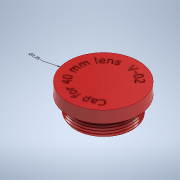
# Autodesk Inventor part: CapForSvBonyPlosse-40mm-V02
Saved by Autodesk Inventor 2021.1 (Build 251245010, 245A)
## iProperties
Created: 2020-10-08
Part Number: CapForSvBonyPlosse-40mm-V02
Material: PC/ABS Plastic
Document SubType Name: Modeling
Designer: robst
Density: 0.357273 g/cm^3
Appearance: Red
Author: robst
Autodesk Inventor part; units mm, degrees
ref_plane "YZ Plane" through (0, 0, 0) normal (1, 0, 0) x (0, 1, 0)
ref_plane "XZ Plane" through (0, 0, 0) normal (0, 1, 0) x (-1, 0, 0)
ref_plane "XY Plane" through (0, 0, 0) normal (0, 0, 1) x (1, 0, 0)
sketch "Sketch7" plane through (0, 0, 0) normal (0, 0, 1) x (1, 0, 0)
  line L0 (0, 0) -> (23.5712, 0)
  line L1 (23.5712, 0) -> (23.5712, 12.7)
  line L2 (23.5712, 12.7) -> (28.575, 12.7)
  line L3 (28.575, 12.7) -> (28.575, 22.225)
  line L4 (28.575, 22.225) -> (0, 22.225)
  line L5 (23.5712, 0) -> (20.3962, 0)
  line L6 (20.3962, 0) -> (20.3962, 19.05)
  line L7 (20.3962, 19.05) -> (0, 19.05)
  line L8 (0, 22.225) -> (0, 19.05)
  line L9 (0, -4.445) -> (0, 26.67) projected
  dimension "d71" = 9.525
  dimension "d72" = 12.7
  dimension "d73" = 23.5712
  dimension "d78" = 3.175
  dimension "d117" = 20.3962
  dimension "d118" = 28.575
  constraints: 18 end point, 5 perpendicular, 2 vertical, 1 horizontal, 1 point on line
  measures "d71" distance between parallel lines of L4 L2
  measures "d72" distance from line of L2 L0.start
  measures "d73" distance of L0.start L0.end
  measures "d78" distance between parallel lines of L1 L6
  measures "d117" distance between parallel lines of L6 L9
  measures "d118" distance from line of L3 L0.start
revolve "Revolution3" add sketch "Sketch7" angle 360 about axis through (0, -10, 0) along (0, 1, 0) contours L6 L7 L8 L4 L3 L2 L1 L0
sketch "Sketch10" plane through (0, 0, 0) normal (0, 0, 1) x (1, 0, 0)
  line L0 (23.5712, 12.7) -> (23.5712, 0) projected
  line L1 (23.5712, -2.1167) -> (23.5712, -4.0025)
  line L2 (23.5712, -4.0025) -> (22.3266, -3.284)
  line L3 (22.3266, -2.8352) -> (23.5712, -2.1167)
  line L4 (-23.5712, 0) -> (23.5712, 0) projected
  arc A0 (22.3266, -2.8352) -> (22.3266, -3.284) centre (22.4561, -3.0596) ccw
  line L5 (0, -7.3431) -> (0, 16.0405) projected
  point P0 (0, 0)
  dimension "d100" = 60
  dimension "d101" = 2.1167
  dimension "d102" = 0.2591
  dimension "d103" = 22.1971
  constraints: 6 end point, 2 point on circle, 2 tangent, 1 centre point, 1 collinear, 1 equal length, 1 vertical
  measures "d100" angle of L3 L2
  measures "d101" distance from line of L1.start L4
  measures "d102" radius of A0
  measures "d103" distance edge to line of A0 L5
coil "Coil6" sketch "Sketch10" operation cut axis through (0, -10, 0) along (0, 1, 0) pitch 2.1167 turns 8 hand right
sketch "Sketch11" plane through (0, 22.225, 0) normal (0, 1, 0) x (1, 0, 0)
  circle A0 centre (0, 0) radius 20.955 construction
  circle A1 centre (0, 0) radius 28.575 projected
  spline S0 degree 2 poles (12.0651, -13.3596) (12.4681, -12.9769) (13.4081, -12.6015) (13.915, -12.6375) knots 0 0 0 1 2 2 2
  spline S1 degree 2 poles (13.915, -12.6375) (14.4186, -12.6701) (15.4561, -13.2177) (15.9536, -13.7416) knots 0 0 0 1 2 2 2
  spline S2 degree 2 poles (15.9536, -13.7416) (16.4479, -14.2621) (16.9162, -15.2864) (16.9354, -15.8111) knots 0 0 0 1 2 2 2
  spline S3 degree 2 poles (16.9354, -15.8111) (16.9516, -16.3258) (16.5507, -17.2622) (16.131, -17.6609) knots 0 0 0 1 2 2 2
  spline S4 degree 2 poles (16.131, -17.6609) (15.9228, -17.8586) (15.4993, -18.1458) (15.3002, -18.2455) knots 0 0 0 1 2 2 2
  spline S5 degree 2 poles (15.3002, -18.2455) (15.1244, -18.3294) (14.7277, -18.4699) (14.5198, -18.5268) knots 0 0 0 1 2 2 2
  line L0 (14.5198, -18.5268) -> (13.8883, -17.8618)
  line L1 (13.8883, -17.8618) -> (13.932, -17.8204)
  spline S6 degree 2 poles (13.932, -17.8204) (14.0697, -17.8174) (14.4766, -17.7886) (14.7273, -17.723) knots 0 0 0 1 2 2 2
  spline S7 degree 2 poles (14.7273, -17.723) (14.968, -17.6604) (15.446, -17.4172) (15.6878, -17.1875) knots 0 0 0 1 2 2 2
  spline S8 degree 2 poles (15.6878, -17.1875) (15.9531, -16.9356) (16.2193, -16.2676) (16.1996, -15.8904) knots 0 0 0 1 2 2 2
  spline S9 degree 2 poles (16.1996, -15.8904) (16.1733, -15.513) (15.7589, -14.6866) (15.3793, -14.287) knots 0 0 0 1 2 2 2
  spline S10 degree 2 poles (15.3793, -14.287) (14.9743, -13.8605) (14.1858, -13.4405) (13.8069, -13.398) knots 0 0 0 1 2 2 2
  spline S11 degree 2 poles (13.8069, -13.398) (13.4377, -13.359) (12.7732, -13.5941) (12.5113, -13.8428) knots 0 0 0 1 2 2 2
  spline S12 degree 2 poles (12.5113, -13.8428) (12.2729, -14.0693) (11.9781, -14.5727) (11.9032, -14.8099) knots 0 0 0 1 2 2 2
  spline S13 degree 2 poles (11.9032, -14.8099) (11.835, -15.0408) (11.7823, -15.4358) (11.7791, -15.5602) knots 0 0 0 1 2 2 2
  line L2 (11.7791, -15.5602) -> (11.7388, -15.5984)
  line L3 (11.7388, -15.5984) -> (11.1137, -14.9402)
  spline S14 degree 2 poles (11.1137, -14.9402) (11.1907, -14.7457) (11.3209, -14.3985) (11.4411, -14.1821) knots 0 0 0 1 2 2 2
  spline S15 degree 2 poles (11.4411, -14.1821) (11.5651, -13.9495) (11.8166, -13.5956) (12.0651, -13.3596) knots 0 0 0 1 2 2 2
  spline S16 degree 2 poles (8.4215, -16.5515) (8.466, -16.4517) (8.6094, -16.104) (8.6959, -15.975) knots 0 0 0 1 2 2 2
  spline S17 degree 2 poles (8.6959, -15.975) (8.8107, -15.7926) (9.0682, -15.5239) (9.3501, -15.3638) knots 0 0 0 1 2 2 2
  spline S18 degree 2 poles (9.3501, -15.3638) (9.5797, -15.2335) (10.0928, -15.1711) (10.3391, -15.239) knots 0 0 0 1 2 2 2
  spline S19 degree 2 poles (10.3391, -15.239) (10.575, -15.3074) (11.0124, -15.6555) (11.1542, -15.9052) knots 0 0 0 1 2 2 2
  spline S20 degree 2 poles (11.1542, -15.9052) (11.3737, -16.2918) (11.3585, -17.0248) (11.0933, -17.3831) knots 0 0 0 1 2 2 2
  spline S21 degree 2 poles (11.0933, -17.3831) (10.8615, -17.7064) (10.0695, -18.3) (9.5901, -18.6095) knots 0 0 0 1 2 2 2
  line L4 (9.5901, -18.6095) -> (9.6587, -18.7303)
  spline S22 degree 2 poles (9.6587, -18.7303) (9.7822, -18.9478) (10.0683, -19.1421) (10.2326, -19.15) knots 0 0 0 1 2 2 2
  spline S23 degree 2 poles (10.2326, -19.15) (10.3969, -19.1579) (10.7707, -19.0096) (10.9559, -18.9044) knots 0 0 0 1 2 2 2
  spline S24 degree 2 poles (10.9559, -18.9044) (11.1734, -18.7809) (11.6882, -18.3182) (11.9113, -18.0264) knots 0 0 0 1 2 2 2
  line L5 (11.9113, -18.0264) -> (11.9475, -18.0058)
  line L6 (11.9475, -18.0058) -> (12.3111, -18.6461)
  spline S25 degree 2 poles (12.3111, -18.6461) (12.1654, -18.7928) (11.5856, -19.2818) (11.2675, -19.4625) knots 0 0 0 1 2 2 2
  spline S26 degree 2 poles (11.2675, -19.4625) (10.8809, -19.682) (10.2847, -19.8608) (9.9861, -19.8226) knots 0 0 0 1 2 2 2
  spline S27 degree 2 poles (9.9861, -19.8226) (9.6938, -19.7862) (9.2157, -19.4133) (9.0167, -19.0629) knots 0 0 0 1 2 2 2
  line L7 (9.0167, -19.0629) -> (7.5691, -16.5136)
  line L8 (7.5691, -16.5136) -> (8.1974, -16.1569)
  line L9 (8.1974, -16.1569) -> (8.4215, -16.5515)
  line L10 (8.7188, -17.0751) -> (9.3065, -18.1101)
  spline S28 degree 2 poles (9.3065, -18.1101) (9.5206, -17.9619) (10.1624, -17.5069) (10.3392, -17.3213) knots 0 0 0 1 2 2 2
  spline S29 degree 2 poles (10.3392, -17.3213) (10.5455, -17.103) (10.691, -16.5996) (10.5309, -16.3177) knots 0 0 0 1 2 2 2
  spline S30 degree 2 poles (10.5309, -16.3177) (10.348, -15.9955) (9.8003, -15.8751) (9.4539, -16.0718) knots 0 0 0 1 2 2 2
  spline S31 degree 2 poles (9.4539, -16.0718) (9.1599, -16.2387) (8.8207, -16.7669) (8.7188, -17.0751) knots 0 0 0 1 2 2 2
  spline S32 degree 2 poles (3.8265, -20.0891) (3.5259, -19.0575) (4.1537, -17.5529) (4.9051, -17.334) knots 0 0 0 1 2 2 2
  spline S33 degree 2 poles (4.9051, -17.334) (5.2119, -17.2446) (5.7247, -17.2496) (6.012, -17.3251) knots 0 0 0 1 2 2 2
  line L11 (6.012, -17.3251) -> (5.5094, -15.5999)
  line L12 (5.5094, -15.5999) -> (6.203, -15.3978)
  line L13 (6.203, -15.3978) -> (7.8443, -21.0314)
  line L14 (7.8443, -21.0314) -> (7.1506, -21.2335)
  line L15 (7.1506, -21.2335) -> (7.025, -20.8022)
  spline S34 degree 2 poles (7.025, -20.8022) (6.8357, -21.113) (6.295, -21.6082) (5.926, -21.7157) knots 0 0 0 1 2 2 2
  spline S35 degree 2 poles (5.926, -21.7157) (5.219, -21.9217) (4.1011, -21.0318) (3.8265, -20.0891) knots 0 0 0 1 2 2 2
  spline S36 degree 2 poles (4.519, -19.8005) (4.725, -20.5075) (5.4008, -21.1548) (5.9032, -21.0084) knots 0 0 0 1 2 2 2
  spline S37 degree 2 poles (5.9032, -21.0084) (6.1967, -20.9229) (6.6716, -20.5) (6.8566, -20.2242) knots 0 0 0 1 2 2 2
  line L16 (6.8566, -20.2242) -> (6.1752, -17.8854)
  spline S38 degree 2 poles (6.1752, -17.8854) (5.8664, -17.8354) (5.4511, -17.8503) (5.2021, -17.9228) knots 0 0 0 1 2 2 2
  spline S39 degree 2 poles (5.2021, -17.9228) (4.6641, -18.0796) (4.2988, -19.0446) (4.519, -19.8005) knots 0 0 0 1 2 2 2
  line L17 (-2.494, -23.284) -> (-2.457, -23.2856)
  spline S40 degree 2 poles (-2.457, -23.2856) (-2.3615, -23.327) (-2.0035, -23.408) (-1.8601, -23.4145) knots 0 0 0 1 2 2 2
  spline S41 degree 2 poles (-1.8601, -23.4145) (-1.4067, -23.4349) (-0.9998, -23.0452) (-0.9756, -22.5085) knots 0 0 0 1 2 2 2
  line L18 (-0.9756, -22.5085) -> (-0.9692, -22.3651)
  line L19 (-0.9692, -22.3651) -> (-2.1628, -22.3114)
  line L20 (-2.1628, -22.3114) -> (-2.136, -21.7146)
  line L21 (-2.136, -21.7146) -> (-0.9654, -21.7672)
  line L22 (-0.9654, -21.7672) -> (-0.7995, -18.0798)
  line L23 (-0.7995, -18.0798) -> (-0.0778, -18.1123)
  line L24 (-0.0778, -18.1123) -> (-0.2437, -21.7997)
  line L25 (-0.2437, -21.7997) -> (0.2421, -21.8216)
  line L26 (0.2421, -21.8216) -> (0.2153, -22.4184)
  line L27 (0.2153, -22.4184) -> (-0.2705, -22.3965)
  line L28 (-0.2705, -22.3965) -> (-0.277, -22.54)
  spline S42 degree 2 poles (-0.277, -22.54) (-0.3115, -23.308) (-1.0926, -24.0795) (-1.7866, -24.0483) knots 0 0 0 1 2 2 2
  spline S43 degree 2 poles (-1.7866, -24.0483) (-1.9856, -24.0393) (-2.3677, -23.9804) (-2.5238, -23.9456) knots 0 0 0 1 2 2 2
  line L29 (-2.5238, -23.9456) -> (-2.494, -23.284)
  spline S44 degree 2 poles (-6.5916, -19.234) (-6.3384, -18.1803) (-5.0492, -17.2755) (-4.2027, -17.4789) knots 0 0 0 1 2 2 2
  spline S45 degree 2 poles (-4.2027, -17.4789) (-3.3336, -17.6878) (-2.623, -19.1112) (-2.8675, -20.1289) knots 0 0 0 1 2 2 2
  spline S46 degree 2 poles (-2.8675, -20.1289) (-3.1186, -21.1737) (-4.4234, -22.0842) (-5.261, -21.883) knots 0 0 0 1 2 2 2
  spline S47 degree 2 poles (-5.261, -21.883) (-6.1076, -21.6795) (-6.8437, -20.2833) (-6.5916, -19.234) knots 0 0 0 1 2 2 2
  spline S48 degree 2 poles (-5.8666, -19.4083) (-6.0614, -20.2188) (-5.6608, -21.1486) (-5.116, -21.2795) knots 0 0 0 1 2 2 2
  spline S49 degree 2 poles (-5.116, -21.2795) (-4.5711, -21.4105) (-3.7873, -20.7653) (-3.5925, -19.9547) knots 0 0 0 1 2 2 2
  spline S50 degree 2 poles (-3.5925, -19.9547) (-3.4032, -19.1667) (-3.8028, -18.2133) (-4.3477, -18.0824) knots 0 0 0 1 2 2 2
  spline S51 degree 2 poles (-4.3477, -18.0824) (-4.888, -17.9525) (-5.674, -18.6067) (-5.8666, -19.4083) knots 0 0 0 1 2 2 2
  line L30 (-10.2887, -19.0566) -> (-10.255, -19.0721)
  spline S52 degree 2 poles (-10.255, -19.0721) (-10.189, -19.128) (-10.0288, -19.2119) (-9.9152, -19.2642) knots 0 0 0 1 2 2 2
  spline S53 degree 2 poles (-9.9152, -19.2642) (-9.6501, -19.3861) (-9.0219, -19.3948) (-8.6818, -19.276) knots 0 0 0 1 2 2 2
  line L31 (-8.6818, -19.276) -> (-7.4098, -16.5119)
  line L32 (-7.4098, -16.5119) -> (-6.7535, -16.814)
  line L33 (-6.7535, -16.814) -> (-8.5463, -20.7098)
  line L34 (-8.5463, -20.7098) -> (-9.2026, -20.4078)
  line L35 (-9.2026, -20.4078) -> (-8.9354, -19.8272)
  spline S54 degree 2 poles (-8.9354, -19.8272) (-9.4402, -19.9824) (-10.0945, -19.9973) (-10.3469, -19.8812) knots 0 0 0 1 2 2 2
  spline S55 degree 2 poles (-10.3469, -19.8812) (-10.4479, -19.8347) (-10.545, -19.7798) (-10.6023, -19.7382) knots 0 0 0 1 2 2 2
  line L36 (-10.6023, -19.7382) -> (-10.2887, -19.0566)
  line L37 (-15.2706, -13.1552) -> (-14.7785, -13.6256)
  line L38 (-14.7785, -13.6256) -> (-13.4217, -12.2061)
  line L39 (-13.4217, -12.2061) -> (-12.8894, -12.7149)
  line L40 (-12.8894, -12.7149) -> (-14.2461, -14.1344)
  line L41 (-14.2461, -14.1344) -> (-12.4215, -15.8784)
  line L42 (-12.4215, -15.8784) -> (-12.9783, -16.4609)
  line L43 (-12.9783, -16.4609) -> (-16.8615, -16.8239)
  line L44 (-16.8615, -16.8239) -> (-17.3704, -16.3375)
  line L45 (-17.3704, -16.3375) -> (-15.2041, -14.0709)
  line L46 (-15.2041, -14.0709) -> (-15.6962, -13.6005)
  line L47 (-15.6962, -13.6005) -> (-15.2706, -13.1552)
  line L48 (-14.6717, -14.5797) -> (-16.2141, -16.1934)
  line L49 (-16.2141, -16.1934) -> (-13.2823, -15.9077)
  line L50 (-13.2823, -15.9077) -> (-14.6717, -14.5797)
  spline S56 degree 2 poles (-18.6083, -9.8076) (-17.3156, -8.9751) (-15.6207, -8.9467) (-15.1167, -9.7294) knots 0 0 0 1 2 2 2
  spline S57 degree 2 poles (-15.1167, -9.7294) (-14.6052, -10.5237) (-15.3606, -12.0623) (-16.626, -12.8772) knots 0 0 0 1 2 2 2
  spline S58 degree 2 poles (-16.626, -12.8772) (-17.9265, -13.7147) (-19.6136, -13.7381) (-20.1202, -12.9515) knots 0 0 0 1 2 2 2
  spline S59 degree 2 poles (-20.1202, -12.9515) (-20.6292, -12.1611) (-19.8621, -10.615) (-18.6083, -9.8076) knots 0 0 0 1 2 2 2
  spline S60 degree 2 poles (-16.6127, -9.6902) (-16.9104, -9.7497) (-17.6926, -10.1433) (-18.1871, -10.4617) knots 0 0 0 1 2 2 2
  spline S61 degree 2 poles (-18.1871, -10.4617) (-18.6816, -10.7802) (-19.3596, -11.3269) (-19.5422, -11.5823) knots 0 0 0 1 2 2 2
  spline S62 degree 2 poles (-19.5422, -11.5823) (-19.7248, -11.8376) (-19.7597, -12.3393) (-19.5867, -12.608) knots 0 0 0 1 2 2 2
  spline S63 degree 2 poles (-19.5867, -12.608) (-19.4137, -12.8767) (-18.9374, -13.0602) (-18.6192, -12.9985) knots 0 0 0 1 2 2 2
  spline S64 degree 2 poles (-18.6192, -12.9985) (-18.3112, -12.9378) (-17.5184, -12.5265) (-17.0473, -12.2231) knots 0 0 0 1 2 2 2
  spline S65 degree 2 poles (-17.0473, -12.2231) (-16.5411, -11.8971) (-15.9037, -11.3985) (-15.7041, -11.1267) knots 0 0 0 1 2 2 2
  spline S66 degree 2 poles (-15.7041, -11.1267) (-15.5151, -10.8728) (-15.4696, -10.3533) (-15.6501, -10.0729) knots 0 0 0 1 2 2 2
  spline S67 degree 2 poles (-15.6501, -10.0729) (-15.8207, -9.8081) (-16.2969, -9.6246) (-16.6127, -9.6902) knots 0 0 0 1 2 2 2
  line L51 (-18.2123, -0.4307) -> (-20.6709, -0.7732)
  spline S68 degree 2 poles (-20.6709, -0.7732) (-20.9645, -0.8141) (-21.4581, -0.9296) (-21.5854, -1.0222) knots 0 0 0 1 2 2 2
  spline S69 degree 2 poles (-21.5854, -1.0222) (-21.7266, -1.1166) (-21.8344, -1.4169) (-21.8005, -1.66) knots 0 0 0 1 2 2 2
  spline S70 degree 2 poles (-21.8005, -1.66) (-21.7699, -1.8802) (-21.4289, -2.347) (-21.135, -2.5773) knots 0 0 0 1 2 2 2
  spline S71 degree 2 poles (-21.135, -2.5773) (-21.0714, -2.5638) (-20.8938, -2.5297) (-20.7745, -2.5131) knots 0 0 0 1 2 2 2
  line L52 (-20.7745, -2.5131) -> (-17.9765, -2.1233)
  line L53 (-17.9765, -2.1233) -> (-17.8768, -2.8388)
  line L54 (-17.8768, -2.8388) -> (-20.3354, -3.1813)
  spline S72 degree 2 poles (-20.3354, -3.1813) (-20.629, -3.2222) (-21.1226, -3.3378) (-21.25, -3.4303) knots 0 0 0 1 2 2 2
  spline S73 degree 2 poles (-21.25, -3.4303) (-21.3911, -3.5248) (-21.4989, -3.8251) (-21.465, -4.0682) knots 0 0 0 1 2 2 2
  spline S74 degree 2 poles (-21.465, -4.0682) (-21.4331, -4.2975) (-21.0732, -4.7664) (-20.8152, -4.9736) knots 0 0 0 1 2 2 2
  line L55 (-20.8152, -4.9736) -> (-17.641, -4.5314)
  line L56 (-17.641, -4.5314) -> (-17.5413, -5.247)
  line L57 (-17.5413, -5.247) -> (-21.7888, -5.8387)
  line L58 (-21.7888, -5.8387) -> (-21.8885, -5.1232)
  line L59 (-21.8885, -5.1232) -> (-21.4207, -5.058)
  spline S75 degree 2 poles (-21.4207, -5.058) (-21.7394, -4.8172) (-22.1235, -4.3095) (-22.1695, -3.9793) knots 0 0 0 1 2 2 2
  spline S76 degree 2 poles (-22.1695, -3.9793) (-22.2219, -3.6031) (-21.959, -2.9727) (-21.5902, -2.767) knots 0 0 0 1 2 2 2
  spline S77 degree 2 poles (-21.5902, -2.767) (-21.9979, -2.4918) (-22.4551, -1.9289) (-22.505, -1.5711) knots 0 0 0 1 2 2 2
  spline S78 degree 2 poles (-22.505, -1.5711) (-22.5433, -1.2959) (-22.4362, -0.8227) (-22.2666, -0.6307) knots 0 0 0 1 2 2 2
  spline S79 degree 2 poles (-22.2666, -0.6307) (-22.0975, -0.4342) (-21.5458, -0.1656) (-21.11, -0.1049) knots 0 0 0 1 2 2 2
  line L60 (-21.11, -0.1049) -> (-18.312, 0.2849)
  line L61 (-18.312, 0.2849) -> (-18.2123, -0.4307)
  line L62 (-17.1923, 6.0248) -> (-19.6136, 6.572)
  spline S80 degree 2 poles (-19.6136, 6.572) (-19.9027, 6.6374) (-20.4053, 6.7035) (-20.5571, 6.6619) knots 0 0 0 1 2 2 2
  spline S81 degree 2 poles (-20.5571, 6.6619) (-20.7225, 6.6233) (-20.9294, 6.3804) (-20.9835, 6.141) knots 0 0 0 1 2 2 2
  spline S82 degree 2 poles (-20.9835, 6.141) (-21.0325, 5.9241) (-20.8783, 5.367) (-20.6845, 5.0478) knots 0 0 0 1 2 2 2
  spline S83 degree 2 poles (-20.6845, 5.0478) (-20.6203, 5.038) (-20.4421, 5.0073) (-20.3246, 4.9807) knots 0 0 0 1 2 2 2
  line L63 (-20.3246, 4.9807) -> (-17.569, 4.3579)
  line L64 (-17.569, 4.3579) -> (-17.7283, 3.6532)
  line L65 (-17.7283, 3.6532) -> (-20.1496, 4.2004)
  spline S84 degree 2 poles (-20.1496, 4.2004) (-20.4387, 4.2658) (-20.9413, 4.3319) (-21.0932, 4.2903) knots 0 0 0 1 2 2 2
  spline S85 degree 2 poles (-21.0932, 4.2903) (-21.2586, 4.2517) (-21.4654, 4.0088) (-21.5195, 3.7694) knots 0 0 0 1 2 2 2
  spline S86 degree 2 poles (-21.5195, 3.7694) (-21.5706, 3.5435) (-21.3993, 2.9778) (-21.231, 2.6928) knots 0 0 0 1 2 2 2
  line L66 (-21.231, 2.6928) -> (-18.1051, 1.9863)
  line L67 (-18.1051, 1.9863) -> (-18.2643, 1.2816)
  line L68 (-18.2643, 1.2816) -> (-22.4474, 2.227)
  line L69 (-22.4474, 2.227) -> (-22.2881, 2.9317)
  line L70 (-22.2881, 2.9317) -> (-21.8273, 2.8276)
  spline S87 degree 2 poles (-21.8273, 2.8276) (-22.0406, 3.1654) (-22.2208, 3.7759) (-22.1472, 4.1012) knots 0 0 0 1 2 2 2
  spline S88 degree 2 poles (-22.1472, 4.1012) (-22.0635, 4.4716) (-21.5951, 4.9687) (-21.1774, 5.031) knots 0 0 0 1 2 2 2
  spline S89 degree 2 poles (-21.1774, 5.031) (-21.4618, 5.4324) (-21.6909, 6.1204) (-21.6112, 6.4728) knots 0 0 0 1 2 2 2
  spline S90 degree 2 poles (-21.6112, 6.4728) (-21.55, 6.7438) (-21.2828, 7.1487) (-21.0563, 7.2685) knots 0 0 0 1 2 2 2
  spline S91 degree 2 poles (-21.0563, 7.2685) (-20.8288, 7.3927) (-20.2177, 7.4493) (-19.7886, 7.3523) knots 0 0 0 1 2 2 2
  line L71 (-19.7886, 7.3523) -> (-17.033, 6.7295)
  line L72 (-17.033, 6.7295) -> (-17.1923, 6.0248)
  line L73 (-14.8611, 10.3342) -> (-15.2617, 9.733)
  line L74 (-15.2617, 9.733) -> (-20.2299, 13.0427)
  line L75 (-20.2299, 13.0427) -> (-19.8294, 13.644)
  line L76 (-19.8294, 13.644) -> (-14.8611, 10.3342)
  spline S92 degree 2 poles (-12.9413, 12.5152) (-13.6429, 11.7637) (-15.257, 11.7246) (-16.0357, 12.4515) knots 0 0 0 1 2 2 2
  spline S93 degree 2 poles (-16.0357, 12.4515) (-16.8008, 13.1657) (-16.959, 14.815) (-16.3554, 15.4617) knots 0 0 0 1 2 2 2
  spline S94 degree 2 poles (-16.3554, 15.4617) (-16.0836, 15.7528) (-15.494, 16.045) (-15.1597, 16.0434) knots 0 0 0 1 2 2 2
  spline S95 degree 2 poles (-15.1597, 16.0434) (-14.8223, 16.0452) (-14.1368, 15.7411) (-13.761, 15.3903) knots 0 0 0 1 2 2 2
  line L77 (-13.761, 15.3903) -> (-13.4733, 15.1216)
  line L78 (-13.4733, 15.1216) -> (-15.4991, 12.9516)
  spline S96 degree 2 poles (-15.4991, 12.9516) (-14.954, 12.4428) (-13.8632, 12.4508) (-13.4081, 12.9383) knots 0 0 0 1 2 2 2
  spline S97 degree 2 poles (-13.4081, 12.9383) (-13.2469, 13.1109) (-13.0119, 13.5188) (-12.9464, 13.7111) knots 0 0 0 1 2 2 2
  spline S98 degree 2 poles (-12.9464, 13.7111) (-12.8814, 13.9165) (-12.8165, 14.2234) (-12.8107, 14.3383) knots 0 0 0 1 2 2 2
  line L79 (-12.8107, 14.3383) -> (-12.7822, 14.3688)
  line L80 (-12.7822, 14.3688) -> (-12.2067, 13.8315)
  spline S99 degree 2 poles (-12.2067, 13.8315) (-12.2548, 13.7054) (-12.4056, 13.3266) (-12.4763, 13.1899) knots 0 0 0 1 2 2 2
  spline S100 degree 2 poles (-12.4763, 13.1899) (-12.5745, 12.9964) (-12.7644, 12.7048) (-12.9413, 12.5152) knots 0 0 0 1 2 2 2
  spline S101 degree 2 poles (-14.3565, 14.9831) (-14.5761, 15.1755) (-14.9697, 15.3782) (-15.1537, 15.3915) knots 0 0 0 1 2 2 2
  spline S102 degree 2 poles (-15.1537, 15.3915) (-15.3575, 15.4108) (-15.7514, 15.2399) (-15.9505, 15.0267) knots 0 0 0 1 2 2 2
  spline S103 degree 2 poles (-15.9505, 15.0267) (-16.1465, 14.8168) (-16.2961, 14.4053) (-16.288, 14.1697) knots 0 0 0 1 2 2 2
  spline S104 degree 2 poles (-16.288, 14.1697) (-16.2734, 13.9342) (-16.0859, 13.5311) (-15.9019, 13.3277) knots 0 0 0 1 2 2 2
  line L81 (-15.9019, 13.3277) -> (-14.3565, 14.9831)
  line L82 (-8.5849, 16.0221) -> (-9.187, 15.6228)
  line L83 (-9.187, 15.6228) -> (-10.5384, 17.6608)
  spline S105 degree 2 poles (-10.5384, 17.6608) (-10.7022, 17.9079) (-11.03, 18.3017) (-11.184, 18.383) knots 0 0 0 1 2 2 2
  spline S106 degree 2 poles (-11.184, 18.383) (-11.3469, 18.4695) (-11.6964, 18.4267) (-11.9203, 18.2782) knots 0 0 0 1 2 2 2
  spline S107 degree 2 poles (-11.9203, 18.2782) (-12.1441, 18.1298) (-12.4602, 17.5757) (-12.5599, 17.2317) knots 0 0 0 1 2 2 2
  line L84 (-12.5599, 17.2317) -> (-10.7888, 14.5607)
  line L85 (-10.7888, 14.5607) -> (-11.3909, 14.1614)
  line L86 (-11.3909, 14.1614) -> (-13.761, 17.7356)
  line L87 (-13.761, 17.7356) -> (-13.1589, 18.1349)
  line L88 (-13.1589, 18.1349) -> (-12.8952, 17.7373)
  spline S108 degree 2 poles (-12.8952, 17.7373) (-12.7863, 18.1596) (-12.4341, 18.7599) (-12.1408, 18.9544) knots 0 0 0 1 2 2 2
  spline S109 degree 2 poles (-12.1408, 18.9544) (-11.6159, 19.3025) (-10.5608, 19.0019) (-10.1231, 18.3419) knots 0 0 0 1 2 2 2
  line L89 (-10.1231, 18.3419) -> (-8.5849, 16.0221)
  spline S110 degree 2 poles (-6.5495, 16.7616) (-6.9513, 16.6065) (-7.7303, 16.5539) (-8.006, 16.5864) knots 0 0 0 1 2 2 2
  line L90 (-8.006, 16.5864) -> (-8.2979, 17.3425)
  line L91 (-8.2979, 17.3425) -> (-8.2634, 17.3558)
  spline S111 degree 2 poles (-8.2634, 17.3558) (-8.1503, 17.3201) (-7.8536, 17.246) (-7.6241, 17.2303) knots 0 0 0 1 2 2 2
  spline S112 degree 2 poles (-7.6241, 17.2303) (-7.4239, 17.2133) (-6.9624, 17.2525) (-6.7421, 17.3376) knots 0 0 0 1 2 2 2
  spline S113 degree 2 poles (-6.7421, 17.3376) (-6.5823, 17.3993) (-6.2434, 17.6146) (-6.1803, 17.7084) knots 0 0 0 1 2 2 2
  spline S114 degree 2 poles (-6.1803, 17.7084) (-6.0867, 17.8389) (-6.0462, 18.068) (-6.1196, 18.2581) knots 0 0 0 1 2 2 2
  spline S115 degree 2 poles (-6.1196, 18.2581) (-6.2113, 18.4957) (-6.5656, 18.6419) (-6.93, 18.5955) knots 0 0 0 1 2 2 2
  spline S116 degree 2 poles (-6.93, 18.5955) (-7.0713, 18.5757) (-7.5194, 18.502) (-7.7149, 18.4811) knots 0 0 0 1 2 2 2
  spline S117 degree 2 poles (-7.7149, 18.4811) (-8.2246, 18.4382) (-8.8529, 18.831) (-9.0047, 19.2242) knots 0 0 0 1 2 2 2
  spline S118 degree 2 poles (-9.0047, 19.2242) (-9.2149, 19.7686) (-8.6603, 20.7622) (-7.9863, 21.0224) knots 0 0 0 1 2 2 2
  spline S119 degree 2 poles (-7.9863, 21.0224) (-7.6536, 21.1509) (-6.9163, 21.247) (-6.6389, 21.2101) knots 0 0 0 1 2 2 2
  line L92 (-6.6389, 21.2101) -> (-6.3603, 20.4886)
  line L93 (-6.3603, 20.4886) -> (-6.3949, 20.4753)
  spline S120 degree 2 poles (-6.3949, 20.4753) (-6.7342, 20.5825) (-7.4567, 20.5766) (-7.7807, 20.4515) knots 0 0 0 1 2 2 2
  spline S121 degree 2 poles (-7.7807, 20.4515) (-8.1134, 20.323) (-8.4629, 19.8653) (-8.3545, 19.5845) knots 0 0 0 1 2 2 2
  spline S122 degree 2 poles (-8.3545, 19.5845) (-8.256, 19.3296) (-7.8887, 19.1884) (-7.5563, 19.2275) knots 0 0 0 1 2 2 2
  spline S123 degree 2 poles (-7.5563, 19.2275) (-7.3944, 19.2453) (-6.9928, 19.311) (-6.7714, 19.3419) knots 0 0 0 1 2 2 2
  spline S124 degree 2 poles (-6.7714, 19.3419) (-6.2873, 19.3997) (-5.6395, 19.0591) (-5.4677, 18.6141) knots 0 0 0 1 2 2 2
  spline S125 degree 2 poles (-5.4677, 18.6141) (-5.3676, 18.3549) (-5.3938, 17.8185) (-5.5274, 17.5733) knots 0 0 0 1 2 2 2
  spline S126 degree 2 poles (-5.5274, 17.5733) (-5.6707, 17.3144) (-6.1391, 16.9201) (-6.5495, 16.7616) knots 0 0 0 1 2 2 2
  line L94 (5.4025, 23.3099) -> (2.7123, 17.8971)
  line L95 (2.7123, 17.8971) -> (1.8995, 18.003)
  line L96 (1.8995, 18.003) -> (0.686, 23.9244)
  line L97 (0.686, 23.9244) -> (1.4943, 23.8191)
  line L98 (1.4943, 23.8191) -> (2.4516, 18.9072)
  line L99 (2.4516, 18.9072) -> (4.6355, 23.4098)
  line L100 (4.6355, 23.4098) -> (5.4025, 23.3099)
  line L101 (7.754, 18.7391) -> (5.7142, 19.4581)
  line L102 (5.7142, 19.4581) -> (5.9451, 20.1133)
  line L103 (5.9451, 20.1133) -> (7.9849, 19.3943)
  line L104 (7.9849, 19.3943) -> (7.754, 18.7391)
  spline S127 degree 2 poles (12.2654, 17.0886) (11.4808, 15.7662) (9.9772, 14.9835) (9.1766, 15.4585) knots 0 0 0 1 2 2 2
  spline S128 degree 2 poles (9.1766, 15.4585) (8.3641, 15.9406) (8.3524, 17.6546) (9.1204, 18.949) knots 0 0 0 1 2 2 2
  spline S129 degree 2 poles (9.1204, 18.949) (9.9096, 20.2794) (11.4086, 21.0541) (12.2131, 20.5767) knots 0 0 0 1 2 2 2
  spline S130 degree 2 poles (12.2131, 20.5767) (13.0217, 20.097) (13.0263, 18.3711) (12.2654, 17.0886) knots 0 0 0 1 2 2 2
  spline S131 degree 2 poles (10.5324, 16.0919) (10.7722, 16.2782) (11.2961, 16.9797) (11.5962, 17.4856) knots 0 0 0 1 2 2 2
  spline S132 degree 2 poles (11.5962, 17.4856) (11.8963, 17.9914) (12.2586, 18.7835) (12.3078, 19.0935) knots 0 0 0 1 2 2 2
  spline S133 degree 2 poles (12.3078, 19.0935) (12.3571, 19.4035) (12.1642, 19.868) (11.8894, 20.0311) knots 0 0 0 1 2 2 2
  spline S134 degree 2 poles (11.8894, 20.0311) (11.6146, 20.1941) (11.1065, 20.1455) (10.8493, 19.9481) knots 0 0 0 1 2 2 2
  spline S135 degree 2 poles (10.8493, 19.9481) (10.6009, 19.7562) (10.0755, 19.034) (9.7895, 18.5521) knots 0 0 0 1 2 2 2
  spline S136 degree 2 poles (9.7895, 18.5521) (9.4823, 18.0343) (9.1349, 17.3034) (9.0778, 16.9711) knots 0 0 0 1 2 2 2
  spline S137 degree 2 poles (9.0778, 16.9711) (9.0221, 16.6595) (9.2136, 16.1743) (9.5003, 16.0042) knots 0 0 0 1 2 2 2
  spline S138 degree 2 poles (9.5003, 16.0042) (9.7712, 15.8435) (10.2793, 15.8921) (10.5324, 16.0919) knots 0 0 0 1 2 2 2
  line L105 (13.904, 11.723) -> (11.3771, 14.1798)
  line L106 (11.3771, 14.1798) -> (11.942, 14.7609)
  spline S139 degree 2 poles (11.942, 14.7609) (12.4629, 14.7518) (13.4094, 14.7553) (13.8904, 14.785) knots 0 0 0 1 2 2 2
  spline S140 degree 2 poles (13.8904, 14.785) (14.859, 14.8445) (15.8015, 15.1296) (16.1211, 15.4583) knots 0 0 0 1 2 2 2
  spline S141 degree 2 poles (16.1211, 15.4583) (16.289, 15.631) (16.4346, 15.9933) (16.419, 16.1699) knots 0 0 0 1 2 2 2
  spline S142 degree 2 poles (16.419, 16.1699) (16.4034, 16.3466) (16.2317, 16.6749) (16.079, 16.8235) knots 0 0 0 1 2 2 2
  spline S143 degree 2 poles (16.079, 16.8235) (15.9329, 16.9655) (15.563, 17.183) (15.372, 17.2589) knots 0 0 0 1 2 2 2
  spline S144 degree 2 poles (15.372, 17.2589) (15.2106, 17.3254) (14.8656, 17.4025) (14.754, 17.4205) knots 0 0 0 1 2 2 2
  line L107 (14.754, 17.4205) -> (14.7241, 17.4496)
  line L108 (14.7241, 17.4496) -> (15.2923, 18.034)
  spline S145 degree 2 poles (15.2923, 18.034) (15.5424, 17.9524) (16.3082, 17.5243) (16.5805, 17.2595) knots 0 0 0 1 2 2 2
  spline S146 degree 2 poles (16.5805, 17.2595) (17.155, 16.701) (17.2117, 15.4638) (16.708, 14.9458) knots 0 0 0 1 2 2 2
  spline S147 degree 2 poles (16.708, 14.9458) (16.4723, 14.7034) (15.9656, 14.4081) (15.6981, 14.3323) knots 0 0 0 1 2 2 2
  spline S148 degree 2 poles (15.6981, 14.3323) (15.4241, 14.2498) (14.793, 14.1787) (14.469, 14.1643) knots 0 0 0 1 2 2 2
  spline S149 degree 2 poles (14.469, 14.1643) (13.9356, 14.1339) (12.7138, 14.1462) (12.3534, 14.1542) knots 0 0 0 1 2 2 2
  line L109 (12.3534, 14.1542) -> (14.3657, 12.1978)
  line L110 (14.3657, 12.1978) -> (13.904, 11.723)
  dimension "d121" = 7.62
  constraints: 1 centre point, 1 coincident, 1 other
  measures "d121" radial gap between concentric circles of A0 A1
extrude "Extrusion1" cut sketch "Sketch11" against normal blind 1.905 contours S0 S1 S2 S3 S4 S5 L0 L1 S6 S7 S8 S9 S10 S11 S12 S13 L2 L3 S14 S15 | S16 S17 S18 S19 S20 S21 L4 S22 S23 S24 L5 L6 S25 S26 S27 L7 L8 L9 | S32 S33 L11 L12 L13 L14 L15 S34 S35 | L17 S40 S41 L18 L19 L20 L21 L22 L23 L24 L25 L26 L27 L28 S42 S43 L29 | S44 S45 S46 S47 | L30 S52 S53 L31 L32 L33 L34 L35 S54 S55 L36 | L37 L38 L39 L40 L41 L42 L43 L44 L45 L46 L47 | S56 S57 S58 S59 | L51 S68 S69 S70 S71 L52 L53 L54 S72 S73 S74 L55 L56 L57 L58 L59 S75 S76 S77 S78 S79 L60 L61 | L62 S80 S81 S82 S83 L63 L64 L65 S84 S85 S86 L66 L67 L68 L69 L70 S87 S88 S89 S90 S91 L71 L72 | L73 L74 L75 L76 | S92 S93 S94 S95 L77 L78 S96 S97 S98 L79 L80 S99 S100 | L82 L83 S105 S106 S107 L84 L85 L86 L87 L88 S108 S109 L89 | S110 L90 L91 S111 S112 S113 S114 S115 S116 S117 S118 S119 L92 L93 S120 S121 S122 S123 S124 S125 S126 | L94 L95 L96 L97 L98 L99 L100 | L101 L102 L103 L104 | S127 S128 S129 S130 | L105 L106 S139 S140 S141 S142 S143 S144 L107 L108 S145 S146 S147 S148 S149 L109 L110
equation "\"d72\" = caseHeightAboveLens"
equation "\"d73\" = a1MajorRadius"
equation "\"d78\" = wallThickness"
equation "\"d118\" = capExteriorRadius"
equation "\"d100\" = threadAngle"
equation "\"d101\" = pitch"
equation "\"d102\" = a1RootRadius"
equation "\"d103\" = a1MinorRadius"
equation "\"d104\" = pitch"
equation "\"baseDiameter\" = 31.75"
equation "\"baseRadius\" = 0.5 * baseDiameter"
equation "\"baseHeight\" = 25.4"
equation "\"middleDiameter\" = 34.29"
equation "\"middleRadius\" = 0.5 * middleDiameter"
equation "\"middleTopDiameter\" = 34.798"
equation "\"middleTopRadius\" = 0.5 * middleTopDiameter"
equation "\"middleHeight\" = 18.542"
equation "\"middleTopHeight\" = 30.734"
equation "\"topBaseDiameter\" = 34.798"
equation "\"topHeightDiameter\" = 40.894"
equation "\"topBaseRadius\" = 0.5 * topBaseDiameter"
equation "\"topHeightRadius\" = 0.5 * topHeightDiameter"
equation "\"topHeight\" = 7.62"
equation "\"d9\" = caseBottomThickness"
equation "\"wallThickness\" = 3.175"
equation "\"caseBottomThickness\" = 4.7625"
equation "\"caseHeightAboveLens\" = 12.7"
equation "\"baseWallThickness\" = 2.032"
equation "\"baseInteriorHeight\" = 15.24"
equation "\"interiorRadius\" = 0.5 * interiorDiameter"
equation "\"outsideRadius\" = interiorRadius + wallThickness"
equation "\"outsideDiameter\" = 2 * outsideRadius"
equation "\"textRingDiameter\" = 0.75 * outsideDiameter"
equation "\"b2MajorDiameterMax\" = 41.275"
equation "\"b2MajorRadiusMax\" = 0.5 * b2MajorDiameterMax"
equation "\"a1MinorDiameter\" = 44.39412"
equation "\"a1MinorRadius\" = 0.5 * a1MinorDiameter"
equation "\"a1MajorDiameter\" = 47.1424"
equation "\"a1MajorRadius\" = 0.5 * a1MajorDiameter"
equation "\"a1RootRadius\" = 0.25908"
equation "\"topThickness\" = 9.525"
equation "\"threadAngle\" = 60deg"
equation "\"capExteriorDiameter\" = 57.15"
equation "\"capExteriorRadius\" = 0.5 * capExteriorDiameter"
equation "\"pitch\" = 2.116667"
equation "\"interiorDiameter\" = 41.275"
body "Solid3"
